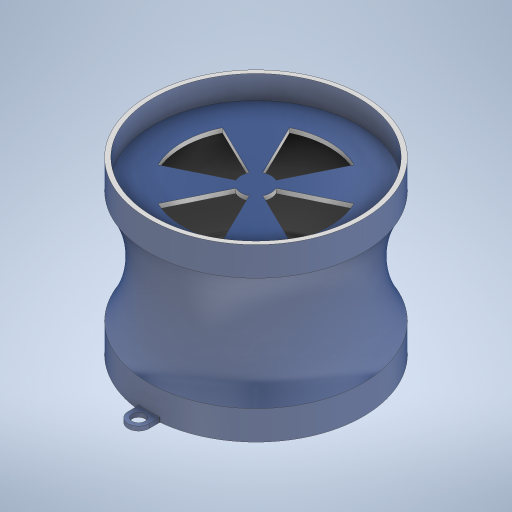
# Autodesk Inventor part: acoplamento_ventoinha1
Saved by Autodesk Inventor 2023 (Build 270158000, 158)
## iProperties
Created: 2023-08-08
Part Number: acoplamento_ventoinha1
Material: Genérico
Document SubType Name: Modeling
Designer: azeve
Density: 1 g/cm^3
Appearance: Padrão
Author: azeve
Autodesk Inventor part; units mm, degrees
ref_plane "YZ Plane" through (0, 0, 0) normal (1, 0, 0) x (0, 1, 0)
ref_plane "XZ Plane" through (0, 0, 0) normal (0, 1, 0) x (-1, 0, 0)
sketch "Esboço1" plane through (0, 0, 0) normal (0, 0, 1) x (1, 0, 0)
  line L0 (25.0389, 40) -> (25.0389, 33.2076)
  line L1 (25.0389, 0) -> (25.0389, 6.7924)
  arc A0 (25.0389, 33.2076) -> (25.0389, 6.7924) centre (48.5809, 20) ccw
  line L2 (24.0389, 0) -> (24.0389, 6.5336)
  line L3 (24.0009, 34.5359) -> (24.0009, 39.0029)
  line L4 (24.0009, 40) -> (25.0389, 40)
  line L5 (24.0389, 33.4664) -> (5.7012, 33.4664)
  line L6 (5.6632, 34.5359) -> (24.0009, 34.5359)
  line L7 (24.0009, 39.0029) -> (24.0009, 40)
  line L8 (5.6632, 34.5359) -> (4.6632, 34.5359)
  line L9 (5.7012, 33.4664) -> (4.7012, 33.4664)
  line L10 (25.0389, 0) -> (24.0389, 0)
  line L11 (24.0009, 34.5359) -> (0.0009, 34.5359)
  line L12 (4.7012, 33.4664) -> (0.0389, 33.4664)
  line L13 (0.0009, 34.5359) -> (0.0009, -0.006)
  line L14 (0.0009, 6.5336) -> (0.0009, 7.5336)
  line L15 (0.0009, 6.5336) -> (0.0009, 7.5336)
  line L16 (0.0009, 6.5336) -> (0.0009, 7.5336)
  line L17 (0.0009, 6.5336) -> (0.0009, 7.5336)
  line L18 (0.0009, 34.5359) -> (0.0009, 33.4664)
  line L19 (0.0389, 33.4664) -> (0.0009, 33.4664)
  line L20 (22.7806, 9.1373) -> (0.0009, 9.1373)
  line L21 (0.0009, 8.062) -> (23.2602, 8.062)
  line L22 (23.5161, 7.5336) -> (24.0389, 6.5336)
  arc A1 (24.0389, 33.4664) -> (22.7806, 9.1373) centre (48.5809, 20) ccw
  arc A2 (23.2602, 8.062) -> (23.5161, 7.5336) centre (48.5809, 20) ccw
  line L23 (0.0009, 9.1373) -> (0.0009, 8.062)
  line L24 (0.0009, 8.062) -> (0.0009, 7.062)
  point P0 (0, 0)
  point P1 (0, 0)
  point P2 (0.0199, 33.4664)
  dimension "d16" = 24.3291
  dimension "d17" = 1.0695
  dimension "d19" = 1
  constraints: 50 end point, 10 point on line, 6 point on circle, 6 vertical, 5 horizontal, 3 centre point, 2 perpendicular, 1 collinear, 1 midpoint
  measures "d16" distance of L20.end point (0.02, 33.466)
  measures "d17" distance of L18.end L11.end
  measures "d19" distance of L21.start L24.end
revolve "Revolução1" add sketch "Esboço1" angle 360 about axis through (0.0009, 34.5359, 0) along (0, -1, 0) contours L0 A0 L1 L10 L2 L22 A2 L21 L13 L20 A1 L5 L9 L12 L19 L11 L8 L6 L3 L7 L4
sketch "Esboço2" plane through (0.0009, 8.062, 0) normal (0, -1, 0) x (1, 0, 0)
  point P0 (-0.0009, 0)
sketch "Esboço3" plane through (0.0009, 34.5359, 0) normal (0, 1, 0) x (1, 0, 0)
  circle A0 centre (-0.0009, 0) radius 3.5
  circle A1 centre (-0.0009, 0) radius 17.1056
  line L0 (-0.0009, 0) -> (-7.5211, 15.3639)
  line L1 (-0.0009, 0) -> (-0.0009, 6.0664)
  line L2 (-0.0009, 0) -> (7.5193, 15.3639)
  line L3 (-0.0009, 0) -> (-15.3648, -7.5202)
  line L4 (-0.0009, 0) -> (-15.3648, 7.5202)
  line L5 (-0.0009, 0) -> (7.5193, -15.3639)
  line L6 (-0.0009, 0) -> (-7.5211, -15.3639)
  line L7 (-0.0009, 0) -> (15.3629, 7.5202)
  line L8 (-0.0009, 0) -> (15.3629, -7.5202)
  point P0 (-3.1445, 1.5387)
  point P1 (-3.1445, -1.5387)
  point P2 (3.1427, -1.5387)
  point P3 (3.1427, 1.5387)
  point P4 (-1.5396, -3.1436)
  point P5 (1.5378, -3.1436)
  point P6 (1.5378, 3.1436)
  point P7 (-1.5396, 3.1436)
  dimension "d1" = 7
  dimension "d4" = 360
  constraints: 18 end point, 2 coincident, 1 centre point, 1 symmetric about line, 1 vertical, 24 other
  measures "d1" diameter of A0
extrude "Extrusão1" cut sketch "Esboço3" against normal blind 10 contours A0 L7 A1 L8 | A0 L0 A1 L2 | L5 A1 L6 A0 | L3 A1 L4 A0
sketch "Esboço4" plane through (0.0009, 8.062, 0) normal (0, -1, 0) x (1, 0, 0)
  circle A0 centre (-0.0009, 0) radius 1.5
  circle A1 centre (-0.0009, 6.6683) radius 1.5
  line L0 (-0.0009, 0) -> (-5.2667, 0)
  circle A2 centre (-0.0009, -6.6683) radius 1.5
  dimension "d8" = 3
  dimension "d9" = 3
  constraints: 3 centre point, 2 end point, 1 coincident, 1 horizontal, 1 symmetric about line, 1 other
  measures "d8" diameter of A0
  measures "d9" diameter of A1
extrude "Extrusão2" cut sketch "Esboço4" against normal blind 10
ref_plane "Plano de trabalho1" through (0.0009, 0, 0) normal (0, -1, 0) x (1, 0, 0)
sketch "Esboço5" plane through (0.0009, 0, 0) normal (0, -1, 0) x (1, 0, 0)
  circle A0 centre (0, 0) radius 25.038 projected
  line L0 (0, 25.038) -> (0, 27.459) construction
  line L1 (-2.4513, 25.038) -> (-2.4513, 27.459)
  line L2 (2.4513, 27.459) -> (2.4513, 25.038)
  arc A1 (2.4513, 27.459) -> (-2.4513, 27.459) centre (0, 27.459) ccw
  line L3 (-7.3697, 0) -> (-12.5067, 0)
  circle A2 centre (0, 27.459) radius 1.4892
  line L4 (-2.4513, -25.038) -> (-2.4513, -27.459)
  line L5 (2.4513, -27.459) -> (2.4513, -25.038)
  arc A3 (-2.4513, -27.459) -> (2.4513, -27.459) centre (0, -27.459) ccw
  circle A4 centre (0, -27.459) radius 1.4892
  arc A5 (-2.4513, 25.038) -> (-2.4484, 24.918) centre (0, 25.038) ccw
  arc A6 (2.4484, 24.918) -> (2.4513, 25.038) centre (0, 25.038) ccw
  arc A7 (2.4513, -25.038) -> (2.4484, -24.918) centre (0, -25.038) ccw
  arc A8 (-2.4484, -24.918) -> (-2.4513, -25.038) centre (0, -25.038) ccw
  point P0 (-0.0009, 0)
  point P1 (0, 26.2485)
  dimension "d15" = 2.9784
  constraints: 17 point on circle, 14 end point, 8 centre point, 7 symmetric about line, 4 tangent, 2 coincident, 1 horizontal, 1 midpoint, 1 parallel, 1 vertical, 2 other
  measures "d15" diameter of A4
extrude "Extrusão3" add sketch "Esboço5" against normal blind 1 contours A0 A5 L1 A1 L2 A6 | A7 L5 A3 L4 A8 A0
